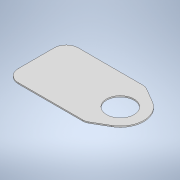
# Autodesk Inventor part: Laser-Pivot-Ringpull
Saved by Autodesk Inventor 2021 (Build 250183000, 183)
## iProperties
Created: 2020-07-21
Part Number: Laser-Pivot-Ringpull
Material: Generic
Document SubType Name: Modeling
Designer: lucas
Density: 1 g/cm^3
Appearance: Default
Project: 4Wire-Laser
Author: lucas
Revision Number: RLS_001
Autodesk Inventor part; units mm, degrees
ref_plane "YZ Plane" through (0, 0, 0) normal (1, 0, 0) x (0, 1, 0)
ref_plane "XZ Plane" through (0, 0, 0) normal (0, 1, 0) x (-1, 0, 0)
ref_plane "XY Plane" through (0, 0, 0) normal (0, 0, 1) x (1, 0, 0)
sketch "Sketch1" plane through (0, 0, 0) normal (0, 1, 0) x (-1, 0, 0)
  circle A0 centre (0, 0) radius 5.7
  arc A1 (0, 9) -> (0, -9) centre (0, 0) ccw construction
  line L0 (0, 9) -> (12.65, 9) construction
  line L1 (12.65, 9) -> (12.65, -9) construction
  line L2 (0, 0) -> (0, -9) construction
  line L3 (3.0786, -12.5) -> (30, -12.5)
  line L4 (35, -7.5) -> (35, 7.5)
  line L5 (30, 12.5) -> (3.0786, 12.5)
  arc A2 (35, 7.5) -> (30, 12.5) centre (30, 7.5) ccw
  arc A3 (30, -12.5) -> (35, -7.5) centre (30, -7.5) ccw
  arc A4 (-4.9268, 8.4715) -> (-4.9268, -8.4715) centre (0, 0) ccw
  line L6 (1.0676, -11.9578) -> (-4.9268, -8.4715)
  line L7 (1.0676, 11.9578) -> (-4.9268, 8.4715)
  arc A5 (1.0676, -11.9578) -> (3.0786, -12.5) centre (3.0786, -8.5) ccw
  arc A6 (3.0786, 12.5) -> (1.0676, 11.9578) centre (3.0786, 8.5) ccw
  point P0 (35, -12.5)
  point P1 (35, 12.5)
  point P2 (2, -12.5)
  point P3 (2, 12.5)
  dimension "d0" = 11.4
  dimension "d1" = 9
  dimension "d2" = 12.65
  dimension "d5" = 25
  dimension "d6" = 5
  dimension "d10" = 25
  dimension "d11" = 19.6
  dimension "d12" = 4
  constraints: 16 end point, 12 point on circle, 10 tangent, 7 centre point, 7 point on line, 3 coincident, 3 perpendicular, 2 equal radius, 2 vertical, 1 horizontal
  measures "d0" diameter of A0
  measures "d1" radius of A1
  measures "d2" distance of L0.start L0.end
  measures "d5" distance of point (35, -12.5) point (35, 12.5)
  measures "d6" radius of A2
  measures "d10" distance between parallel lines of L5 L3
  measures "d11" diameter of A4
  measures "d12" radius of A5
extrude "Extrusion1" add sketch "Sketch1" along normal blind 0.5
body "Solid1"
